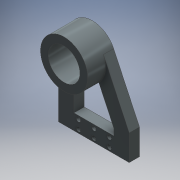
# Autodesk Inventor part: chassi_front_right
Saved by Autodesk Inventor 2016 (Build 200138000, 138)
## iProperties
Created: 2017-01-01
Part Number: chassi_front_right
Material: Generic
Document SubType Name: Modeling
Designer: hesaon
Density: 1 g/cm^3
Appearance: Default
Author: hesaon
Autodesk Inventor part; units mm, degrees
ref_plane "YZ Plane" through (0, 0, 0) normal (1, 0, 0) x (0, 1, 0)
ref_plane "XZ Plane" through (0, 0, 0) normal (0, 1, 0) x (-1, 0, 0)
ref_plane "XY Plane" through (0, 0, 0) normal (0, 0, 1) x (1, 0, 0)
sketch "Sketch1" plane through (0, 0, 0) normal (0, 1, 0) x (-1, 0, 0)
  line L0 (-55, -52.5) -> (-24.8972, 11.6781)
  line L1 (-55, -82.5) -> (-55, -52.5)
  line L2 (27.5, 0) -> (27.5, -82.5)
  line L3 (9.5, -64.5) -> (-37, -64.5)
  line L4 (9.5, -64.5) -> (9.5, -25.807)
  line L5 (-37, -64.5) -> (-37, -56.5118)
  arc A0 (27.5, 0) -> (-24.8972, 11.6781) centre (0, 0) ccw
  arc A1 (-19.56, -19.3302) -> (9.5, -25.807) centre (0, 0) ccw
  circle A2 centre (0, 7) radius 6.25
  circle A3 centre (15.5, 0) radius 1.6
  circle A4 centre (7.75, 13.4234) radius 1.6
  circle A5 centre (-7.75, 13.4234) radius 1.6
  circle A6 centre (-15.5, 0) radius 1.6
  circle A7 centre (-7.75, -13.4234) radius 1.6
  circle A8 centre (7.75, -13.4234) radius 1.6
  line L6 (-19.56, -19.3302) -> (-37, -56.5118)
  line L7 (27.5, -82.5) -> (-55, -82.5)
  dimension "d12" = 18
  dimension "d13" = 82.5
  dimension "d14" = 12.5
  dimension "d15" = 7
  dimension "d16" = 3.2
  dimension "d17" = 15.5
  dimension "d20" = 360
  dimension "d22" = 30
  dimension "d23" = 27.5
  dimension "d24" = 18
  dimension "d25" = 27.5
  dimension "d26" = 27.5
  dimension "d27" = 27.5
  dimension "d29" = 18
  dimension "d30" = 18
  dimension "d31" = 82.5
  dimension "d32" = 82.5
  constraints: 16 end point, 9 centre point, 4 point on circle, 3 vertical, 2 horizontal, 2 tangent, 1 horizontal alignment, 1 parallel, 1 vertical alignment, 13 other
  measures "d12" distance from line of L1 L3.end
  measures "d13" distance of L2.end L1.start
  measures "d14" diameter of A2
  measures "d15" distance of point (0, 0) A2.centre
  measures "d16" diameter of A3
  measures "d17" distance of point (0, 0) A3.centre
  measures "d22" distance of L1.start L0.start
  measures "d23" radius of A0
  measures "d24" distance between parallel lines of L4 L2
  measures "d25" radius of A1
  measures "d26" distance of L2.start point (0, 0)
  measures "d27" distance from line of L0 point (0, 0)
  measures "d29" distance between parallel lines of L0 L6
  measures "d30" distance between parallel lines of L7 L3
  measures "d31" distance from line of point (0, 0) L7
  measures "d32" distance of L2.end L2.start
extrude "Extrusion1" add sketch "Sketch1" along normal blind 6
sketch "Sketch2" plane through (0, 0, 0) normal (0, -1, 0) x (1, 0, 0)
  arc A0 (24.8972, 11.6781) -> (-27.5, 0) centre (0, 0) ccw projected
  circle A1 centre (0, 0) radius 27.5
  circle A2 centre (0, 0) radius 18.5
  dimension "d35" = 37
  constraints: 2 centre point, 2 coincident, 1 concentric
  measures "d35" diameter of A2
extrude "Extrusion2" add sketch "Sketch2" along normal blind 27
sketch "Sketch5" plane through (0, 0, 0) normal (0, -1, 0) x (1, 0, 0)
  line L0 (-27.5, -82.5) -> (-27.5, 0) projected
  line L1 (-27.5, 0) -> (-27.5, -82.5)
  line L2 (55, -82.5) -> (-27.5, -82.5) projected
  line L3 (-27.5, -82.5) -> (55, -82.5)
  line L4 (55, -82.5) -> (55, -52.5)
  line L5 (24.8972, 11.6781) -> (55, -52.5) projected
  line L6 (55, -52.5) -> (24.8972, 11.6781)
  line L7 (37, -56.5118) -> (19.56, -19.3302) projected
  line L8 (19.56, -19.3302) -> (37, -56.5118)
  line L9 (37, -64.5) -> (37, -56.5118) projected
  line L10 (37, -56.5118) -> (37, -64.5)
  line L11 (-9.5, -25.807) -> (-9.5, -64.5) projected
  line L12 (37, -64.5) -> (-9.5, -64.5)
  line L13 (-9.5, -64.5) -> (-9.5, -25.807)
  arc A0 (19.56, -19.3302) -> (24.8972, 11.6781) centre (0, 0) ccw
  arc A1 (-27.5, 0) -> (-9.5, -25.807) centre (0, 0) ccw
  constraints: 16 end point, 4 collinear, 4 point on circle, 3 perpendicular, 2 centre point, 1 coincident, 1 vertical
extrude "Extrusion5" add sketch "Sketch5" along normal blind 6
sketch "Sketch7" plane through (0, -6, 0) normal (0, -1, 0) x (1, 0, 0)
  circle A0 centre (-4.25, -68.5) radius 2.5
  circle A1 centre (13.75, -68.5) radius 2.5
  line L0 (-9.5, -64.5) -> (-9.5, -25.807) projected
  line L1 (37, -64.5) -> (-9.5, -64.5) projected
  circle A2 centre (-4.25, -78.5) radius 2.5
  circle A3 centre (13.75, -78.5) radius 2.5
  circle A4 centre (31.75, -68.5) radius 2.5
  circle A5 centre (31.75, -78.5) radius 2.5
  line L2 (37, -56.5118) -> (37, -64.5) projected
  point P0 (0, 0)
  dimension "d63" = 5
  dimension "d64" = 5
  dimension "d65" = 18
  dimension "d66" = 5.25
  dimension "d67" = 4
  dimension "d68" = 5
  dimension "d69" = 5
  dimension "d70" = 10
  dimension "d72" = 18
  dimension "d73" = 5
  dimension "d74" = 5
  dimension "d82" = 18
  constraints: 6 centre point, 4 horizontal alignment, 2 vertical alignment
  measures "d63" diameter of A0
  measures "d64" diameter of A1
  measures "d65" distance of A1.centre A0.centre
  measures "d66" distance from line of A0.centre L0
  measures "d67" distance from line of L1 A0.centre
  measures "d68" diameter of A2
  measures "d69" diameter of A3
  measures "d70" distance of A0.centre A2.centre
  measures "d72" distance of A3.centre A2.centre
  measures "d73" diameter of A4
  measures "d74" diameter of A5
  measures "d82" distance of A3.centre A5.centre
extrude "Extrusion7" cut sketch "Sketch7" against normal up to next
body "Solid1"
